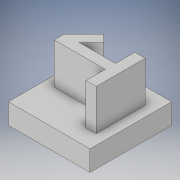
# Autodesk Inventor part: 1
Saved by Autodesk Inventor 2019 (Build 230136000, 136)
## iProperties
Created: 2018-08-09
Part Number: 1
Material: Generic
Document SubType Name: Modeling
Designer: Ge Shi
Density: 1 g/cm^3
Appearance: Default
Author: Ge Shi
Autodesk Inventor part; units mm, degrees
ref_plane "YZ Plane" through (0, 0, 0) normal (1, 0, 0) x (0, 1, 0)
ref_plane "XZ Plane" through (0, 0, 0) normal (0, 1, 0) x (-1, 0, 0)
ref_plane "XY Plane" through (0, 0, 0) normal (0, 0, 1) x (1, 0, 0)
sketch "Sketch1" plane through (0, 0, 0) normal (0, 1, 0) x (-1, 0, 0)
  line L0 (-10, -10) -> (10, -10)
  line L1 (10, -10) -> (10, 10)
  line L2 (10, 10) -> (-10, 10)
  line L3 (-10, 10) -> (-10, -10)
  line L4 (-10, -10) -> (10, 10) construction
  line L5 (10, -10) -> (-10, 10) construction
  point P0 (0, 0)
  dimension "d0" = 20
  dimension "d1" = 20
  constraints: 12 end point, 2 midpoint, 2 parallel, 1 horizontal, 1 perpendicular
  measures "d0" distance of L2.end L1.end
  measures "d1" distance of L0.end L1.end
extrude "Extrusion1" add sketch "Sketch1" against normal blind 5
sketch "Sketch2" plane through (0, 0, 0) normal (0, 1, 0) x (-1, 0, 0)
  line L0 (10, -10) -> (10, 10) projected
  line L1 (-10, 10) -> (-10, -10) projected
  line L2 (14, 0) -> (-14, 0) projected
  line L3 (7.5, 1.25) -> (7.5, -1.25)
  line L4 (7.5, -1.25) -> (2.7322, -6.0178)
  line L5 (2.7322, -6.0178) -> (0.9645, -4.25)
  line L6 (0.9645, -4.25) -> (3.9645, -1.25)
  line L7 (3.9645, -1.25) -> (-5, -1.25)
  line L8 (-5, -1.25) -> (-5, -6)
  line L9 (-5, -6) -> (-7.5, -6)
  line L10 (-7.5, -6) -> (-7.5, 6)
  line L11 (-7.5, 6) -> (-5, 6)
  line L12 (-5, 6) -> (-5, 1.25)
  line L13 (-5, 1.25) -> (7.5, 1.25)
  point P0 (0, 0)
  dimension "d13" = 2.5
  dimension "d14" = 2.5
  dimension "d15" = 2.5
  dimension "d16" = 2.5
  dimension "d17" = 3
  dimension "d18" = 12
  dimension "d19" = 2.5
  dimension "d20" = 2.5
  dimension "d21" = 45
  constraints: 22 end point, 8 perpendicular, 2 point on line, 1 collinear, 1 vertical, 1 other
  measures "d13" distance between parallel lines of L4 L6
  measures "d14" distance between parallel lines of L7 L13
  measures "d15" distance of L3.start L3.end
  measures "d16" distance of L8.end L9.end
  measures "d17" horizontal distance of L5.end L6.end
  measures "d18" distance of L9.end L10.end
  measures "d19" distance between parallel lines of L1 L10
  measures "d20" distance between parallel lines of L0 L3
  measures "d21" angle of L7 L6
extrude "Extrusion2" add sketch "Sketch2" along normal blind 10
body "Solid1"
